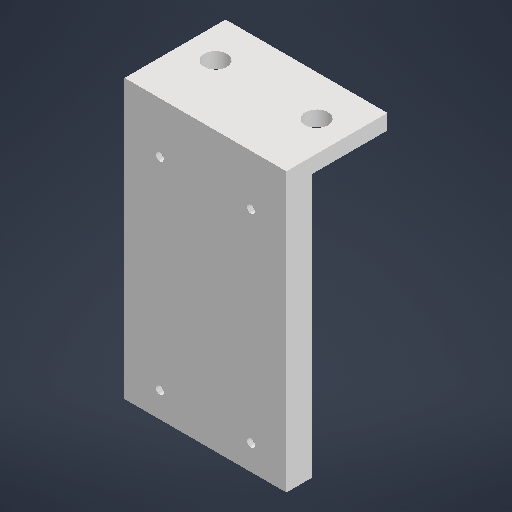
# Autodesk Inventor part: Support
Saved by Autodesk Inventor 2026.1 (Build 301233020, 233B)
## iProperties
Created: 2025-11-07
Part Number: Support
Material: 일반
Document SubType Name: Modeling
Designer: alexi
Density: 1 g/cm^3
Appearance: 기본값
Author: alexi
Autodesk Inventor part; units mm, degrees
ref_plane "YZ Plane" through (0, 0, 0) normal (1, 0, 0) x (0, 1, 0)
ref_plane "XZ Plane" through (0, 0, 0) normal (0, 1, 0) x (-1, 0, 0)
ref_plane "XY Plane" through (0, 0, 0) normal (0, 0, 1) x (1, 0, 0)
ref_plane "작업 평면1" through (0, 0, 0) normal (0, 0, 1) x (1, 0, 0)
sketch "스케치1" plane through (0, 0, 0) normal (0, 0, 1) x (1, 0, 0)
  line L0 (13, -22) -> (-13, -22) construction
  line L1 (13, 22) -> (13, -22) construction
  line L2 (-13, 22) -> (13, 22) construction
  line L3 (-13, -22) -> (-13, 22) construction
  circle A0 centre (9, -20) radius 1.2 construction
  circle A1 centre (9, 20) radius 1.2 construction
  circle A2 centre (-9, -20) radius 1.2 construction
  circle A3 centre (-9, 20) radius 1.2 construction
  line L4 (-16, 30) -> (16, 30)
  line L5 (16, 30) -> (16, -25)
  line L6 (16, -25) -> (-16, -25)
  line L7 (-16, -25) -> (-16, 30)
  point P0 (0, 0)
  dimension "d0" = 3
  dimension "d1" = 8
  dimension "d2" = 3
  dimension "d3" = 3
  constraints: 16 end point, 4 centre point, 3 horizontal, 2 parallel, 2 vertical, 1 perpendicular, 13 other
  measures "d0" distance between parallel lines of L3 L7
  measures "d1" distance between parallel lines of L2 L4
  measures "d2" distance between parallel lines of L5 L1
  measures "d3" distance between parallel lines of L6 L0
extrude "돌출1" add sketch "스케치1" along normal blind 5
sketch "스케치2" plane through (0, 0, 0) normal (0, 0, -1) x (-1, 0, 0)
  line L0 (-13, -22) -> (13, -22) construction
  line L1 (13, -22) -> (13, 22) construction
  line L2 (13, 22) -> (-13, 22) construction
  line L3 (-13, 22) -> (-13, -22) construction
  circle A0 centre (-9, -20) radius 1.2 construction
  circle A1 centre (-9, 20) radius 1.2 construction
  circle A2 centre (9, -20) radius 1.2 construction
  circle A3 centre (9, 20) radius 1.2 construction
  line L4 (1, 16) -> (14, 16)
  line L5 (14, 16) -> (14, -16)
  line L6 (14, -16) -> (1, -16)
  line L7 (1, -16) -> (1, 16)
  line L8 (-16, -25) -> (-16, 30) projected
  line L9 (16, 30) -> (16, -25) projected
  line L10 (-16, 30) -> (16, 30)
  line L11 (16, 30) -> (16, 27)
  line L12 (-16, 27) -> (-16, 30)
  point P0 (0, 0)
  dimension "d6" = 1
  dimension "d7" = 16
  dimension "d8" = 16
  dimension "d9" = 12
  constraints: 22 end point, 4 centre point, 4 horizontal, 3 parallel, 2 perpendicular, 2 vertical, 1 point on line, 13 other
  measures "d6" distance between parallel lines of L5 L1
  measures "d7" distance from line of point (0, 0) L4
  measures "d8" distance from line of L6 point (0, 0)
  measures "d9" distance between parallel lines of L1 L7
extrude "돌출2" cut sketch "스케치2" against normal blind 3
sketch "스케치3" plane through (0, 0, 0) normal (0, 0, -1) x (-1, 0, 0)
  line L0 (-16, -25) -> (-16, 30) projected
  line L1 (-16, 27) -> (16, 27)
  line L2 (16, 30) -> (16, -25) projected
  line L3 (-16, 30) -> (16, 30) projected
  point P0 (0, 0)
  dimension "d13" = 3
  constraints: 2 end point, 2 point on line, 1 horizontal
  measures "d13" distance between parallel lines of L3 L1
extrude "돌출3" add sketch "스케치3" along normal blind 15
sketch "스케치4" plane through (-16, 30, 5) normal (0, 1, 0) x (1, 0, 0)
  point P0 (16, 5)
  point P1 (6, 12)
  point P2 (26, 12)
  dimension "d16" = 20
  dimension "d17" = 10
  dimension "d18" = 7
  dimension "d19" = 7
  measures "d16" distance of point (26, 12) point (6, 12)
  measures "d17" horizontal distance of point (16, 5) point (26, 12)
  measures "d18" vertical distance of point (16, 5) point (6, 12)
  measures "d19" vertical distance of point (16, 5) point (26, 12)
hole "구멍1" at (10, 30, -7) at (-10, 30, -7) direction (0, -1, 0) diameter 4.5 depth 3 tip angle 118
sketch "스케치5" plane through (0, 0, 0) normal (0, 0, -1) x (-1, 0, 0)
  point P0 (0, 0)
  point P1 (-9, 20)
  point P2 (-9, -20)
  point P3 (9, -20)
  point P4 (9, 20)
  constraints: 4 other
hole "구멍2" at (-9, 20, 0) at (9, 20, 0) at (9, -20, 0) at (-9, -20, 0) direction (0, 0, 1) diameter 1.567 depth 5 tip angle 118 thread size "M2x0.4" class "6H" standard "ANSI Metric M Profile"
equation "\"d2\" = d0"
equation "\"d3\" = d0"
equation "\"d8\" = d7"
equation "\"d17\" = 0.5 * d16"
equation "\"d18\" = d19"
